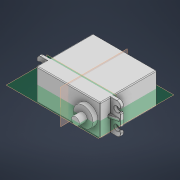
# Autodesk Inventor part: servo_moter
Saved by Autodesk Inventor 2021 (Build 250183000, 183)
## iProperties
Created: 2020-09-30
Part Number: servo_moter
Material: 일반
Document SubType Name: Modeling
Designer: sbahn
Density: 1 g/cm^3
Appearance: 기본값
Author: sbahn
Autodesk Inventor part; units mm, degrees
ref_plane "YZ Plane" through (0, 0, 0) normal (1, 0, 0) x (0, 1, 0)
ref_plane "XZ Plane" through (0, 0, 0) normal (0, 1, 0) x (-1, 0, 0)
ref_plane "XY Plane" through (0, 0, 0) normal (0, 0, 1) x (1, 0, 0)
sketch "스케치1" plane through (0, 0, 0) normal (0, 0, 1) x (1, 0, 0)
  line L0 (0, 0) -> (40.6, 0)
  line L1 (40.6, 0) -> (40.6, 19.8)
  line L2 (40.6, 19.8) -> (0, 19.8)
  line L3 (0, 19.8) -> (0, 0)
  dimension "d0" = 40.6
  dimension "d1" = 19.8
  constraints: 8 end point, 2 parallel, 1 horizontal, 1 perpendicular
  measures "d0" distance of L2.end L1.end
  measures "d1" distance of L1.end L0.end
extrude "돌출1" add sketch "스케치1" along normal blind 38.6
ref_plane "작업 평면1" through (0, 0, 27) normal (0, 0, -1) x (-1, 0, 0)
sketch "스케치2" plane through (0, 0, 27) normal (0, 0, -1) x (-1, 0, 0)
  line L0 (-40.6, 0) -> (-40.6, 19.8) projected
  line L1 (-40.6, 19.8) -> (0, 19.8) projected
  line L2 (0, 19.8) -> (0, 0) projected
  line L3 (0, 0) -> (-40.6, 0) projected
  line L4 (6.4, 19.8) -> (-47, 19.8)
  line L5 (-47, 19.8) -> (-47, 0)
  line L6 (-47, 0) -> (6.4, 0)
  line L7 (6.4, 0) -> (6.4, 19.8)
  line L8 (0, 0) -> (-40.6, 0) projected
  line L9 (-40.6, 19.8) -> (0, 19.8) projected
  line L10 (-20.3, 19.8) -> (-20.3, 34.9429) construction
  dimension "d9" = 53.4
  dimension "d11" = 26.7
  constraints: 10 end point, 2 parallel, 2 point on line, 1 horizontal, 1 midpoint, 1 perpendicular, 1 vertical
  measures "d9" distance between parallel lines of L5 L7
  measures "d11" distance between parallel lines of L10 L5
extrude "돌출2" add sketch "스케치2" against normal blind 2 contours L6 L5 L4 L0 | L2 L4 L7 L6
sketch "스케치4" plane through (0, 0, 29) normal (0, 0, 1) x (1, 0, 0)
  line L0 (-6.4, 19.8) -> (0, 19.8) projected
  line L1 (0, 0) -> (0, 19.8) construction
  line L2 (0, 0) -> (-6.4, 0) construction
  line L3 (-6.4, 0) -> (-6.4, 19.8) construction
  line L4 (-6.4, 19.8) -> (46.9516, 19.8) construction
  line L5 (46.9516, 19.8) -> (46.9516, 0) construction
  line L6 (46.9516, 0) -> (-6.4, 0) construction
  line L7 (-6.4, 0) -> (-6.4, 19.8) construction
  line L8 (-3.9, 15) -> (44.5, 15) construction
  line L9 (44.5, 15) -> (44.5, 4.8) construction
  line L10 (44.5, 4.8) -> (-3.9, 4.8) construction
  line L11 (-3.9, 4.8) -> (-3.9, 15) construction
  line L12 (-6.4, 0) -> (-6.4, 19.8) construction
  line L13 (-6.4, 9.9) -> (-10.8641, 9.9) construction
  line L14 (40.6, 19.8) -> (0, 19.8) construction
  line L15 (20.3, 19.8) -> (20.3, 26.8295)
  circle A0 centre (-3.9, 15) radius 1.75
  line L16 (-8.882, 16.25) -> (-4.7285, 16.25)
  line L17 (-4.7285, 16.25) -> (-4.7285, 13.75)
  line L18 (-4.7285, 13.75) -> (-8.882, 13.75)
  line L19 (-8.882, 13.75) -> (-8.882, 16.25)
  point P0 (-5.1247, 13.75)
  point P1 (-5.1247, 16.25)
  dimension "d23" = 48.4
  dimension "d24" = 24.2
  dimension "d25" = 10.2
  dimension "d26" = 5.1
  dimension "d27" = 3.5
  dimension "d28" = 2.5
  dimension "d29" = 1.25
  constraints: 28 end point, 6 parallel, 4 horizontal, 3 perpendicular, 2 midpoint, 1 centre point, 1 coincident, 1 vertical
  measures "d23" distance of L8.start L8.end
  measures "d24" distance between parallel lines of L15 L11
  measures "d25" distance of L10.end L8.start
  measures "d26" distance between parallel lines of L13 L10
  measures "d27" diameter of A0
  measures "d28" distance of L18.end L16.start
  measures "d29" distance from line of L8.start L16
extrude "돌출4" cut sketch "스케치4" against normal blind 5
fillet "모깎기1" radius 0.5 4 edges at (-5.1247, 16.25, 28) (-5.1247, 13.75, 28) (-6.4, 16.25, 28) (-6.4, 13.75, 28)
pattern_linear "직사각형 패턴1" count 2 spacing 10.2 along (0, -1, 0) of "돌출4"
ref_plane "작업 평면3" through (20.3, 0, 38.6) normal (1, 0, 0) x (0, 0, -1)
mirror "미러1" about plane through (20.3, 0, 38.6) normal (1, 0, 0) of "모깎기1", "돌출4", "직사각형 패턴1"
fillet "모깎기2" radius 2.5 4 edges at (-6.4, 0, 28) (-6.4, 19.8, 28) (47, 19.8, 28) (47, 0, 28)
sketch "스케치5" plane through (0, 0, 38.6) normal (0, 0, 1) x (1, 0, 0)
  line L0 (40.6, 0) -> (40.6, 19.8) projected
  line L1 (40.6, 19.8) -> (0, 19.8) projected
  line L2 (0, 19.8) -> (0, 0) projected
  line L3 (0, 0) -> (40.6, 0) projected
  line L4 (0, 0) -> (0, 19.8) projected
  line L5 (0, 9.9) -> (40.6, 9.9)
  circle A0 centre (32.8, 9.9) radius 6.25
  line L6 (20.3, 9.9) -> (20.3, 4.5969) construction
  dimension "d39" = 12.5
  dimension "d40" = 12.5
  constraints: 4 end point, 3 midpoint, 1 centre point, 1 point on line
  measures "d39" diameter of A0
  measures "d40" distance from line of A0.centre L6
extrude "돌출5" cut sketch "스케치5" against normal blind 3 contours L3 L2 L5 A0 L0 | L5 A0 L2 L1 L0
sketch "스케치6" plane through (32.8, 9.9, 38.6) normal (0, 0, 1) x (1, 0, 0)
  circle A0 centre (0, 0) radius 6.25 projected
  circle A1 centre (0, 0) radius 2.5
  point P0 (-32.8, -9.9)
  dimension "d41" = 5
  constraints: 1 centre point, 1 coincident
  measures "d41" diameter of A1
extrude "돌출6" add sketch "스케치6" along normal blind 5 contours A1
fillet "모깎기3" radius 0.5 8 edges at (0, 19.8, 13.5) (40.6, 19.8, 13.5) (40.6, 0, 13.5) (0, 0, 13.5) (40.6, 19.8, 32.3) (40.6, 0, 32.3) (0, 19.8, 32.3) (0, 0, 32.3)
ref_plane "작업 평면4" through (-3.9, 9.9, 27) normal (0, -1, 0) x (1, 0, 0)
sketch "스케치7" plane through (-3.9, 9.9, 27) normal (0, -1, 0) x (1, 0, 0)
  line L0 (3.9, 2) -> (3.9, 8.6) projected
  line L1 (4.4, 2) -> (0, 2) projected
  line L2 (-1.0999, 2) -> (1.75, 2) projected
  line L3 (-1.6981, 2) -> (3.9, 3.5)
  line L4 (-1.0999, 2) -> (-2.5099, 2)
  point P0 (3.9, -27)
  point P1 (-1.6981, 2)
  dimension "d45" = 15
  dimension "d46" = 1.5
  constraints: 4 end point, 2 point on line, 1 horizontal
  measures "d45" angle of L1 L3
  measures "d46" distance of L0.start L3.end
extrude "돌출7" add sketch "스케치7" along normal mid plane 2
fillet "모깎기4" radius 0.2 2 edges at (-2.799, 8.9, 29.75) (-2.799, 10.9, 29.75)
fillet "모깎기5" radius 0.5 8 edges at (-6.4, 6.05, 28) (-5.1247, 6.05, 28) (-5.1247, 3.55, 28) (-6.4, 3.55, 28) (47, 6.05, 28) (45.7247, 3.55, 28) (45.7247, 6.05, 28) (47, 3.55, 28)
fillet "모깎기6" radius 0.2 40 edges at (-5.6678, 0.7322, 29) (-6.4, 2.775, 29) (-6.2536, 3.4036, 29) (-5.6071, 3.55, 29) (-5.1475, 3.5214, 29) (-2.15, 4.8, 29) (-5.1475, 6.0786, 29) (-5.6071, 6.05, 29) (-6.2536, 6.1964, 29) (-6.4, 9.9, 29) (-6.2536, 13.6036, 29) (-5.6071, 13.75, 29) (-5.1475, 13.7214, 29) (-2.15, 15, 29) (-5.1475, 16.2786, 29) (-5.6071, 16.25, 29) (-6.2536, 16.3964, 29) (-6.4, 17.025, 29) (-5.6678, 19.0678, 29) (-1.7, 19.8, 29) (-1.7, 0, 29) (46.2678, 0.7322, 29) (47, 2.775, 29) (46.8536, 3.4036, 29) (46.2071, 3.55, 29) (45.7475, 3.5214, 29) (42.75, 4.8, 29) (45.7475, 6.0786, 29) (46.2071, 6.05, 29) (46.8536, 6.1964, 29) (47, 9.9, 29) (46.2071, 13.75, 29) (45.7475, 13.7214, 29) (42.75, 15, 29) (45.7475, 16.2786, 29) (46.2071, 16.25, 29) (47, 17.025, 29) (46.2678, 19.0678, 29) (42.3, 19.8, 29) (42.3, 0, 29)
mirror "미러2" about plane through (20.3, 0, 38.6) normal (1, 0, 0) of "돌출7", "모깎기4"
fillet "모깎기7" radius 0.2 5 edges at (0, 8.9586, 30.4394) (0, 9.9, 30.5) (0, 10.8414, 30.4394) (0, 10.9, 29.6465) (0, 8.9, 29.6465)
fillet "모깎기8" radius 0.2 13 edges at (-5.3717, 8.9586, 29) (-5.5981, 9.9, 29) (-5.3717, 10.8414, 29) (-2.5127, 10.9, 29) (-0.0586, 10.9586, 29) (0, 15.2, 29) (0.0257, 19.4581, 29) (0.2716, 19.7448, 28.938) (-0.0586, 8.8414, 29) (0, 4.6, 29) (0.0257, 0.3419, 29) (0.2716, 0.0552, 28.938) (-2.5127, 8.9, 29)
fillet "모깎기9" radius 0.2 5 edges at (40.6, 8.9, 29.6465) (40.6, 9.9, 30.5) (40.6, 10.8414, 30.4394) (40.6, 10.9, 29.6465) (40.6, 8.9586, 30.4394)
fillet "모깎기10" radius 0.2 13 edges at (40.6586, 8.8414, 29) (43.1127, 8.9, 29) (45.9717, 8.9586, 29) (46.1981, 9.9, 29) (45.9717, 10.8414, 29) (43.1127, 10.9, 29) (40.6586, 10.9586, 29) (40.6, 15.2, 29) (40.5743, 19.4581, 29) (40.3284, 19.7448, 28.938) (40.5743, 0.3419, 29) (40.3284, 0.0552, 28.938) (40.6, 4.6, 29)
fillet "모깎기11" radius 0.2 40 edges at (46.2678, 0.7322, 27) (47, 2.775, 27) (46.8536, 3.4036, 27) (46.2071, 3.55, 27) (45.7475, 3.5214, 27) (42.75, 4.8, 27) (45.7475, 6.0786, 27) (46.2071, 6.05, 27) (46.8536, 6.1964, 27) (47, 9.9, 27) (46.2071, 13.75, 27) (45.7475, 13.7214, 27) (42.75, 15, 27) (45.7475, 16.2786, 27) (46.2071, 16.25, 27) (47, 17.025, 27) (46.2678, 19.0678, 27) (42.3, 19.8, 27) (42.3, 0, 27) (-1.7, 0, 27) (-6.4, 2.775, 27) (-6.2536, 3.4036, 27) (-5.6071, 3.55, 27) (-5.1475, 3.5214, 27) (-2.15, 4.8, 27) (-5.1475, 6.0786, 27) (-5.6071, 6.05, 27) (-6.2536, 6.1964, 27) (-6.4, 9.9, 27) (-6.2536, 13.6036, 27) (-5.6071, 13.75, 27) (-5.1475, 13.7214, 27) (-2.15, 15, 27) (-5.1475, 16.2786, 27) (-5.6071, 16.25, 27) (-6.2536, 16.3964, 27) (-6.4, 17.025, 27) (-5.6678, 19.0678, 27) (-1.7, 19.8, 27) (-5.6678, 0.7322, 27)
fillet "모깎기12" radius 0.5 8 edges at (0.1464, 19.6536, 35.6) (20.3, 19.8, 35.6) (40.4536, 19.6536, 35.6) (40.6, 9.9, 35.6) (40.4536, 0.1464, 35.6) (20.3, 0, 35.6) (0.1464, 0.1464, 35.6) (0, 9.9, 35.6)
equation "\"d11\" = 0.5 * d9"
equation "\"d24\" = 0.5 * d23"
equation "\"d26\" = 0.5 * d25"
equation "\"d29\" = 0.5 * d28"
